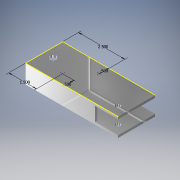
# Autodesk Inventor part: 15102898-16-P-0203
Saved by Autodesk Inventor 2017 (Build 210142000, 142)
## iProperties
Created: 2016-09-30
Part Number: 15102898-16-P-0203
Material: Aluminum 6061
Document SubType Name: Modeling
Designer: gus
Density: 2.7 g/cm^3
Appearance: Aluminum - Flat
Mass: 147.217 g
Surface Area: 355.501 cm^2
Volume: 54.5247 cm^3
Author: gus
Autodesk Inventor part; units mm, degrees
ref_plane "YZ Plane" through (0, 0, 0) normal (1, 0, 0) x (0, 1, 0)
ref_plane "XZ Plane" through (0, 0, 0) normal (0, 1, 0) x (-1, 0, 0)
ref_plane "XY Plane" through (0, 0, 0) normal (0, 0, 1) x (1, 0, 0)
sketch "Sketch1" plane through (0, 0, 0) normal (0, 0, 1) x (1, 0, 0)
  line L0 (0, 0) -> (-127, 0)
  line L1 (-127, 0) -> (-127, 25.4)
  line L2 (-127, 25.4) -> (0, 25.4)
  line L3 (0, 0) -> (0, 3.175)
  line L4 (0, 3.175) -> (-98.425, 3.175)
  line L5 (-98.425, 3.175) -> (-98.425, 22.225)
  line L6 (-98.425, 22.225) -> (0, 22.225)
  line L7 (0, 22.225) -> (0, 25.4)
  dimension "d0" = 127
  dimension "d1" = 25.4
  dimension "d2" = 3.175
  dimension "d3" = 98.425
  dimension "d4" = 19.05
  constraints: 16 end point, 5 perpendicular, 1 horizontal, 1 parallel, 1 point on line, 1 vertical
  measures "d0" distance of L1.end L2.end
  measures "d1" distance of L0.end L1.end
  measures "d2" distance of L0.start L3.end
  measures "d3" distance of L3.end L4.end
  measures "d4" distance of L4.end L5.end
extrude "Extrusion1" add sketch "Sketch1" along normal blind 50.8
sketch "Sketch2" plane through (-127, 25.4, 0) normal (0, 1, 0) x (1, 0, 0)
  circle A0 centre (114.3, -38.1) radius 3.175
  line L0 (127, 0) -> (127, -50.8) projected
  line L1 (127, -50.8) -> (0, -50.8) projected
  line L2 (0, -50.8) -> (127, -50.8) projected
  line L3 (0, -50.8) -> (95.25, -50.8)
  line L4 (95.25, -50.8) -> (95.25, -47.625)
  line L5 (95.25, -47.625) -> (0, -47.625)
  line L6 (0, -47.625) -> (0, -50.8)
  line L7 (127, 0) -> (0, 0) projected
  line L8 (0, -3.175) -> (95.25, -3.175)
  line L9 (95.25, -3.175) -> (95.25, 0)
  line L10 (95.25, 0) -> (0, 0)
  line L11 (0, 0) -> (0, -3.175)
  circle A1 centre (12.7, -25.4) radius 4.7625
  line L12 (0, 0) -> (0, -50.8) projected
  dimension "d7" = 6.35
  dimension "d8" = 12.7
  dimension "d9" = 12.7
  dimension "d12" = 31.75
  dimension "d13" = 3.175
  dimension "d19" = 9.525
  dimension "d20" = 12.7
  dimension "d21" = 25.4
  constraints: 16 end point, 4 parallel, 2 centre point, 2 equal length, 2 horizontal, 2 perpendicular, 2 point on line
  measures "d7" diameter of A0
  measures "d8" distance from line of A0.centre L0
  measures "d9" distance from line of A0.centre L1
  measures "d12" distance between parallel lines of L0 L9
  measures "d13" distance of L8.end L9.end
  measures "d19" diameter of A1
  measures "d20" distance from line of L12 A1.centre
  measures "d21" distance from line of L7 A1.centre
extrude "Extrusion2" cut sketch "Sketch2" against normal blind 50.8 contours A0 | A1
extrude "Extrusion3" add sketch "Sketch2" against normal blind 25.4 contours L9 L8 L11 L7 | L1 L6 L5 L4
sketch "Sketch3" plane through (-127, 0, 0) normal (-1, 0, 0) x (0, 0, 1)
  line L0 (3.175, 22.225) -> (3.175, 3.175) projected
  line L1 (0, 22.225) -> (50.8, 22.225) projected
  line L2 (3.175, 3.175) -> (47.625, 3.175)
  line L3 (47.625, 3.175) -> (47.625, 22.225)
  line L4 (47.625, 22.225) -> (3.175, 22.225)
  line L5 (3.175, 22.225) -> (3.175, 3.175)
  point P0 (0, 0)
  dimension "d16" = 44.45
  constraints: 8 end point, 2 parallel, 1 horizontal, 1 perpendicular, 1 point on line
  measures "d16" distance of L0.end L2.end
extrude "Extrusion4" cut sketch "Sketch3" against normal blind 25.4
sketch "Sketch4" plane through (-127, 25.4, 50.8) normal (0, 1, 0) x (1, 0, 0)
  line L0 (0, 50.8) -> (127, 50.8) projected
  line L1 (127, 0) -> (0, 0) projected
  line L2 (0, 50.8) -> (0, 0) projected
  point P0 (38.1, 12.7)
  point P1 (63.5, 38.1)
  dimension "d22" = 12.7
  dimension "d23" = 12.7
  dimension "d24" = 38.1
  dimension "d25" = 63.5
  measures "d22" distance from line of L0 point (63.5, 38.1)
  measures "d23" distance from line of L1 point (38.1, 12.7)
  measures "d24" distance from line of L2 point (38.1, 12.7)
  measures "d25" distance from line of L2 point (63.5, 38.1)
hole "Hole1" at (-88.9, 25.4, 38.1) at (-63.5, 25.4, 12.7) direction (0, -1, 0) diameter 6.35 end through all
body "Solid1"
